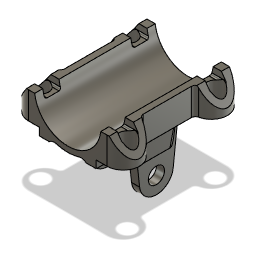
0.883.3680 - Demi-collier à chape - IGTE 21465_204886 (Autodesk Fusion 360 design; units mm, degrees)
Autodesk Fusion 360 part; units mm, degrees
sketch "Sketch1" plane through (0, 0, 0) normal (0, 0, 1) x (1, 0, 0)
  line L0 (0, 0) -> (0, -55) construction
  line L1 (-30.5, 0) -> (-30.5, -55) construction
  line L2 (30.5, 0) -> (30.5, -55) construction
  line L3 (0, 0) -> (100, 0) construction
  line L4 (0, 0) -> (-100, 0) construction
  line L5 (0, 67.5) -> (100, 67.5) construction
  line L6 (0, -67.5) -> (100, -67.5) construction
  line L7 (0, -67.5) -> (-100, -67.5) construction
  line L8 (0, -55) -> (0, -67.5) construction
  line L9 (0, -3) -> (100, -3) construction
  line L10 (0, -3) -> (-100, -3) construction
  line L11 (15, 0) -> (15, -55) construction
  line L12 (15, -55) -> (15, -67.5) construction
  line L13 (-15, 0) -> (-15, -55) construction
  line L14 (-15, -55) -> (-15, -67.5) construction
  line L15 (-15, -67.5) -> (-21, -67.5)
  arc A0 (-24.4164, -3) -> (0, -24.6) centre (0, 0) ccw
  line L16 (-30.5, -3) -> (-28.4422, -3)
  line L17 (28.4422, -3) -> (30.5, -3)
  line L18 (-30.5, -3) -> (-30.5, -23) construction
  line L19 (-30.5, -23) -> (-41, -23)
  line L20 (-41, -23) -> (-41, -18)
  line L21 (-41, -18) -> (-30.5, -3)
  line L22 (-21, -67.5) -> (-21, -22.9991)
  arc A1 (-28.4422, -3) -> (-22.9689, -17.0408) centre (0, 0) ccw
  arc A2 (-8.5119, -27.304) -> (0, -28.6) centre (0, 0) ccw
  arc A3 (-21, -22.9991) -> (-22.9689, -17.0408) centre (-31, -22.9991) ccw
  line L23 (-15, -67.5) -> (-15, -32.0774)
  arc A4 (-8.5119, -27.304) -> (-15, -32.0774) centre (-10, -32.0774) ccw
  line L24 (-24.4164, -3) -> (-28.4422, -3)
  line L25 (-30.5, -23) -> (-21, -23)
  line L26 (15, -67.5) -> (21, -67.5)
  line L27 (15, -55) -> (15, -67.5) construction
  line L28 (21, -67.5) -> (21, -22.9991)
  line L29 (15, -67.5) -> (15, -32.0774)
  arc A5 (15, -32.0774) -> (8.5119, -27.304) centre (10, -32.0774) ccw
  arc A6 (0, -28.6) -> (8.5119, -27.304) centre (0, 0) ccw
  arc A7 (0, -24.6) -> (24.4164, -3) centre (0, 0) ccw
  arc A8 (22.9689, -17.0408) -> (21, -22.9991) centre (31, -22.9991) ccw
  arc A9 (22.9689, -17.0408) -> (28.4422, -3) centre (0, 0) ccw
  line L30 (24.4164, -3) -> (28.4422, -3)
  line L31 (30.5, -3) -> (28.4422, -3)
  line L32 (41, -18) -> (30.5, -3)
  line L33 (41, -23) -> (41, -18)
  line L34 (30.5, -23) -> (41, -23)
  line L35 (30.5, -23) -> (21, -23)
  dimension "d1" = 55
  dimension "d2" = 30.5
  dimension "d3" = 30.5
  dimension "d4" = 100
  dimension "d6" = 67.5
  dimension "d7" = 3
  dimension "d8" = 15
  dimension "d9" = 15
  dimension "d11" = 6
  dimension "d14" = 24.6
  dimension "d15" = 28.6
  dimension "d19" = 20
  dimension "d20" = 10.5
  dimension "d21" = 5
  dimension "d22" = 10
  dimension "d23" = 5
  constraint coincident L0.start L3.start
  constraint symmetric L0 L3.start L4.start
  constraint symmetric L0 L3.end L4.end
  constraint parallel L3 L5
  constraint perpendicular L7 L8
  constraint coincident L9 L17.start
  constraint coincident L10 A0.start
  constraint coincident L10 L16.end
  constraint coincident L10 L16.start
  constraint coincident L1 L16.start
  constraint perpendicular L1 L16
  constraint coincident L9 L17.end
  constraint coincident L2 L17.end
  constraint perpendicular L2 L17
  constraint perpendicular L15 L22
  constraint concentric A1 A2
  constraint tangent L22 A3
  constraint tangent A1 A3
  constraint perpendicular L15 L23
  constraint tangent L23 A4
  constraint tangent A2 A4
  constraint coincident L0 A2.end
  constraint coincident L0 A0.end
  constraint perpendicular L13 L24
  constraint perpendicular L22 L25
  constraint coincident L22 L25.end
  constraint symmetric L0 L13.end L11.end
  constraint symmetric L0 L14.end L12.end
  constraint symmetric L0 L15.end L26.end
  constraint symmetric L0 A0.start A7.end
  constraint symmetric L0 A0 A7
  constraint symmetric L0 L16.end L17.start
  constraint symmetric L0 L16.start L17.end
  constraint symmetric L0 L18.end L34.start
  constraint symmetric L0 L19.end L33.start
  constraint symmetric L0 L20.end L32.start
  constraint symmetric L0 A1 A9
  constraint symmetric L0 A2 A6
  constraint symmetric L0 L22.end L28.end
  constraint symmetric L0 A1.end A8.start
  constraint symmetric L0 A3 A8
  constraint symmetric L0 L23.end L29.end
  constraint symmetric L0 A2.start A5.end
  constraint symmetric L0 A4 A5
  constraint symmetric L0 A2.end A6.start
  constraint symmetric L0 A0.end A7.start
  constraint symmetric L0 L25.end L35.end
  measures "d1" distance of L0.start L0.end
  measures "d4" distance of L0.start L3.end
  measures "d11" distance of L14.end L15.end
  measures "d14" radius of A0
  measures "d15" radius of A1
  measures "d19" distance of L16.start L18.end
  measures "d20" distance of L18.end L19.end
  measures "d21" distance of L19.end L20.end
  measures "d22" radius of A3
  measures "d23" radius of A4
extrude "Extrude1" add sketch "Sketch1" along normal mid plane 89
sketch "Sketch2" plane through (0, 0, 0) normal (1, 0, 0) x (0, 0, -1)
  line L0 (44.5, -3) -> (-44.5, -3) construction
  line L1 (0, 0) -> (0, -110) construction
  line L2 (0, 0) -> (100, 0) construction
  line L3 (0, 0) -> (-100, 0) construction
  line L4 (0, -55) -> (-100, -55) construction
  line L5 (0, -55) -> (100, -55) construction
  circle A0 centre (0, -55) radius 6
  line L6 (-44.5, -67.5) -> (-44.5, -23) construction
  line L7 (-44.5, -23) -> (-44.5, -18) construction
  line L8 (-44.5, -18) -> (-44.5, -3)
  line L9 (44.5, -3) -> (-44.5, -3) construction
  line L10 (44.5, -3) -> (44.5, -18) construction
  line L11 (44.5, -18) -> (44.5, -23) construction
  line L12 (44.5, -23) -> (44.5, -67.5) construction
  line L13 (44.5, -67.5) -> (-44.5, -67.5) construction
  arc A1 (-12.424, -56.3759) -> (12.424, -56.3759) centre (0, -55) ccw
  line L14 (44.5, -27.304) -> (-44.5, -27.304) construction
  line L15 (-44.5, -27.304) -> (-44.5, -28.6)
  line L16 (-44.5, -27.304) -> (44.5, -27.304) construction
  line L17 (44.5, -28.6) -> (44.5, -27.304)
  line L18 (-44.5, -27.304) -> (-44.5, -28.6)
  line L19 (-44.5, -28.6) -> (44.5, -28.6)
  line L20 (-15.5, 0) -> (-15.5, -110) construction
  line L21 (15.5, 0) -> (15.5, -110) construction
  line L22 (15.5, -28.6) -> (12.424, -56.3759)
  line L23 (-15.5, -28.6) -> (-12.424, -56.3759)
  line L24 (44.5, -3) -> (44.5, -28.6)
  line L25 (-44.5, -3) -> (-44.5, -28.6)
  line L26 (37, -9) -> (-31, -9) construction
  line L27 (-32.5, 0) -> (-32.5, -110) construction
  line L28 (32.5, 0) -> (32.5, -110) construction
  line L29 (21.5, -3) -> (32.5, -3)
  line L30 (32.5, -3) -> (44.5, -3) construction
  line L31 (0, -3) -> (9.5, -3)
  line L32 (0, -3) -> (-9.5, -3)
  line L33 (44.5, -28.6) -> (44.5, -67.5)
  line L34 (0, -67.5) -> (44.5, -67.5)
  line L35 (-44.5, -28.6) -> (-44.5, -67.5)
  line L36 (-44.5, -67.5) -> (0, -67.5)
  line L37 (9.5, -3) -> (21.5, -3)
  line L38 (-44.5, -3) -> (-32.5, -3)
  line L39 (-20.5, -3) -> (0, -3)
  line L40 (20.5, -3) -> (0, -3)
  line L41 (-44.5, -9) -> (31, -9) construction
  line L42 (44.5, -3) -> (32.5, -3) construction
  line L43 (32.5, -3) -> (35.5, -3) construction
  line L44 (44.5, -3) -> (-44.5, -3)
  line L45 (44.5, -3) -> (38.5, -3) construction
  line L46 (38.5, -3) -> (38.5, -7.5)
  line L47 (37, -9) -> (28, -9)
  line L48 (26.5, -7.5) -> (26.5, -3)
  arc A2 (37, -9) -> (38.5, -7.5) centre (37, -7.5) ccw
  arc A3 (26.5, -7.5) -> (28, -9) centre (28, -7.5) ccw
  line L49 (-38.5, -3) -> (-38.5, -7.5)
  arc A4 (-38.5, -7.5) -> (-37, -9) centre (-37, -7.5) ccw
  line L50 (-37, -9) -> (-28, -9)
  arc A5 (-28, -9) -> (-26.5, -7.5) centre (-28, -7.5) ccw
  line L51 (-26.5, -7.5) -> (-26.5, -3)
  point P0 (35.5, -9)
  point P1 (23.5, -9)
  point P2 (-35.5, -9)
  point P3 (-23.5, -9)
  point P4 (26.5, -9)
  dimension "d26" = 55
  dimension "d27" = 12
  dimension "d28" = 25
  dimension "d29" = 15.5
  dimension "d30" = 15.5
  dimension "d32" = 6
  dimension "d33" = 32.5
  dimension "d34" = 32.5
  dimension "d40" = 12
  dimension "d56" = 3
  dimension "d57" = 6
  dimension "d58" = 12
  dimension "d61" = 12
  dimension "d63" = 6
  dimension "d66" = 1.5
  dimension "d67" = 1.5
  constraint coincident L1.start L2.start
  constraint perpendicular L0 L1
  constraint perpendicular L1 L2
  constraint symmetric L1 L2.start L3.start
  constraint symmetric L1 L2.end L3.end
  constraint coincident L4.start L5.start
  constraint concentric A0 A1
  constraint coincident L15.end L18.end
  constraint coincident L17.start L19.end
  constraint coincident L21 L22.start
  constraint coincident L19 L22.start
  constraint tangent A1 L22
  constraint coincident L20 L23.start
  constraint coincident L19 L23.start
  constraint tangent A1 L23
  constraint coincident L0.start L9.start
  constraint coincident L0.end L8.end
  constraint coincident L9 L29.start
  constraint coincident L28 L29.end
  constraint coincident L0 L29.end
  constraint coincident L0 L31.end
  constraint midpoint L0 L31.start
  constraint symmetric L1 L31.end L32.end
  constraint symmetric L1 L31.start L32.start
  constraint coincident L12.end L13.start
  constraint midpoint L13 L34.start
  constraint coincident L6.start L13.end
  constraint tangent A1 L36
  constraint coincident L9 L39.start
  constraint symmetric L1 L0.end L0.start
  constraint coincident L41 P2
  constraint perpendicular L0 L48
  constraint coincident L0 L48.end
  constraint tangent L46 A2
  constraint tangent L26 A2
  constraint coincident P4 L47
  constraint coincident P4 L48
  constraint tangent L47 A3
  constraint tangent L48 A3
  constraint symmetric L1 L45.end L49.start
  constraint symmetric L1 L48.end L51.end
  constraint symmetric L1 L46.end L49.end
  constraint symmetric L1 L26.start A4.end
  constraint symmetric L1 A2 A4
  constraint symmetric L1 L47.end L50.end
  constraint symmetric L1 L48.start A5.end
  constraint symmetric L1 A3 A5
  measures "d27" diameter of A0
  measures "d28" diameter of A1
  measures "d32" distance of L9 L26
  measures "d40" distance of L0.end L38.end
  measures "d56" distance of L29.end L43.end
  measures "d57" distance of L43.end P0
  measures "d58" distance of P0 P1
  measures "d61" distance of P2 P3
  measures "d63" distance of L0.start L45.end
  measures "d66" radius of A2
  measures "d67" radius of A3
extrude "Extrude2" cut sketch "Sketch2" along normal through all and the other way through all contours A0 | L38 L44 L49 A4 L50 A5 L51 | A1 L19 L23 L35 L36 | A1 L19 L22 L33 L34 | L29 L44 L46 L47 L48 A2 A3
sketch "Sketch3" plane through (0, 0, 0) normal (0, 1, 0) x (1, 0, 0)
  line L0 (-41, 44.5) -> (-41, -44.5) construction
  line L1 (41, 44.5) -> (41, -44.5) construction
  line L2 (-24.4164, 44.5) -> (24.4164, 44.5) construction
  line L3 (24.4164, 44.5) -> (30.5, 44.5) construction
  line L4 (30.5, 44.5) -> (41, 44.5) construction
  line L5 (-24.4164, 44.5) -> (-30.5, 44.5) construction
  line L6 (-41, 44.5) -> (-30.5, 44.5) construction
  line L7 (-30.5, -44.5) -> (-41, -44.5) construction
  line L8 (-24.4164, -44.5) -> (-30.5, -44.5) construction
  line L9 (24.4164, -44.5) -> (-24.4164, -44.5) construction
  line L10 (30.5, -44.5) -> (24.4164, -44.5) construction
  line L11 (41, -44.5) -> (30.5, -44.5) construction
  line L12 (0, -44.5) -> (0, 44.5) construction
  line L13 (-41, 0) -> (41, 0) construction
  line L14 (29, -44.5) -> (29, -32.5) construction
  line L15 (29, -32.5) -> (41, -32.5) construction
  line L16 (41, -32.5) -> (41, -44.5) construction
  line L17 (29, 32.5) -> (41, 32.5) construction
  line L18 (29, 44.5) -> (29, 32.5) construction
  line L19 (-29, 32.5) -> (-41, 32.5) construction
  line L20 (-29, 44.5) -> (-29, 32.5) construction
  line L21 (-29, -32.5) -> (-41, -32.5) construction
  line L22 (-29, -44.5) -> (-29, -32.5) construction
  line L23 (29, -32.5) -> (29, -20.5) construction
  arc A0 (29, -44.5) -> (31.4, -20.7424) centre (29, -32.5) ccw
  arc A1 (31.4, 20.7424) -> (29, 44.5) centre (29, 32.5) ccw
  line L24 (29, 32.5) -> (29, 20.5) construction
  line L25 (-29, -32.5) -> (-29, -20.5) construction
  arc A2 (-31.4, -20.7424) -> (-29, -44.5) centre (-29, -32.5) ccw
  line L26 (-29, 32.5) -> (-29, 20.5) construction
  arc A3 (-29, 44.5) -> (-31.4, 20.7424) centre (-29, 32.5) ccw
  line L27 (-29, -17.8031) -> (-29, 17.8031)
  line L28 (29, -17.8031) -> (29, 17.8031)
  line L29 (-29, -44.5) -> (29, -44.5)
  line L30 (-29, 44.5) -> (29, 44.5)
  arc A4 (29, -17.8031) -> (31.4, -20.7424) centre (32, -17.8031) ccw
  arc A5 (31.4, 20.7424) -> (29, 17.8031) centre (32, 17.8031) ccw
  arc A6 (-31.4, -20.7424) -> (-29, -17.8031) centre (-32, -17.8031) ccw
  arc A7 (-29, 17.8031) -> (-31.4, 20.7424) centre (-32, 17.8031) ccw
  line L31 (-41, -32.5) -> (-41, 32.5)
  line L32 (41, -32.5) -> (41, 32.5)
  line L33 (41, 32.5) -> (41, 44.5)
  line L34 (29, 44.5) -> (41, 44.5)
  line L35 (-41, 32.5) -> (-41, 44.5)
  line L36 (-29, 44.5) -> (-41, 44.5)
  line L37 (-29, -44.5) -> (-41, -44.5)
  line L38 (-41, -44.5) -> (-41, -32.5)
  line L39 (41, -44.5) -> (41, -32.5)
  line L40 (29, -44.5) -> (41, -44.5)
  line L41 (29, -32.5) -> (32, -32.5)
  circle A8 centre (32, -32.5) radius 6
  circle A9 centre (32, 32.5) radius 6
  circle A10 centre (-32, 32.5) radius 6
  circle A11 centre (-32, -32.5) radius 6
  line L42 (-30.5, 38.5) -> (-24.4164, 38.5)
  dimension "d44" = 12
  dimension "d45" = 12
  dimension "d47" = 3
  dimension "d55" = 12
  constraint midpoint L9 L12.start
  constraint midpoint L2 L12.end
  constraint midpoint L0 L13.start
  constraint midpoint L1 L13.end
  constraint vertical L14
  constraint horizontal L15
  constraint vertical L16
  constraint coincident L1.end L11.start
  constraint symmetric L13 L14.start L18.start
  constraint symmetric L13 L14.end L17.start
  constraint symmetric L13 L15.end L17.end
  constraint symmetric L12 L14.start L22.start
  constraint symmetric L12 L14.end L21.start
  constraint symmetric L12 L15.end L21.end
  constraint symmetric L12 L17.start L19.start
  constraint symmetric L12 L17.end L19.end
  constraint symmetric L12 L18.start L20.start
  constraint coincident L14.end L15.start
  constraint coincident L15.end A0
  constraint perpendicular L15 L23
  constraint symmetric L13 L23.end L24.end
  constraint symmetric L13 A0 A1
  constraint symmetric L12 L23.end L25.end
  constraint symmetric L12 A0 A2
  constraint symmetric L12 L24.end L26.end
  constraint symmetric L12 A1 A3
  constraint tangent L27 A7
  constraint tangent A3 A7
  constraint equal A4 A7
  constraint coincident L1.start L4.end
  constraint coincident L0.start L6.start
  constraint coincident L0.end L7.end
  constraint coincident L41.end A8.centre
  constraint symmetric L13 A8 A9
  constraint symmetric L12 A8 A11
  constraint symmetric L12 A9 A10
  measures "d44" distance of L1.end L15.end
  measures "d45" distance of L1.end L14.start
  measures "d47" radius of A4
  measures "d55" diameter of A8
extrude "Extrude3" cut sketch "Sketch3" along normal through all and the other way through all contours A0 L39 L40 | A0 A1 L28 A4 A5 L32 | A2 L37 L38 | A1 L33 L34 | A2 A3 L27 A6 A7 L31 | A3 L35 L36 | A8 | A9 | A10 | A11
sketch "Sketch4" plane through (0, 0, 0) normal (0, 0, 1) x (1, 0, 0)
  arc A0 (-24.4164, -3) -> (24.4164, -3) centre (0, 0) ccw construction
  arc A1 (-8.5119, -27.304) -> (8.5119, -27.304) centre (0, 0) ccw construction
  line L0 (21, -67.5) -> (21, -56.3759) construction
  line L1 (15, -56.3759) -> (15, -67.5) construction
  line L2 (15, -56.3759) -> (15, -32.0774) construction
  line L3 (15, -56.3759) -> (21, -56.3759) construction
  line L4 (21, -28.6) -> (21, -56.3759) construction
  line L5 (21, -23) -> (29, -23) construction
  line L6 (21, -28.6) -> (21, -23) construction
  line L7 (29, -23) -> (41, -23) construction
  line L8 (29, -3) -> (24.4164, -3) construction
  line L9 (30.5, -3) -> (29, -3) construction
  line L10 (41, -18) -> (30.5, -3) construction
  line L11 (0, 0) -> (0, -83.2034) construction
  circle A2 centre (0, 0) radius 28.6 construction
  line L12 (15, -67.5) -> (21, -67.5) construction
  line L13 (15, -42.5) -> (21, -42.5) construction
  line L14 (21, -42.5) -> (28.0922, -5.3652)
  line L15 (21, -42.5) -> (21, -19.4155)
  arc A3 (21, -19.4155) -> (28.0922, -5.3652) centre (0, 0) ccw
  line L16 (-21, -42.5) -> (-21, -19.4155)
  arc A4 (-28.0922, -5.3652) -> (-21, -19.4155) centre (0, 0) ccw
  line L17 (-21, -42.5) -> (-28.0922, -5.3652)
  dimension "d50" = 25
  constraint coincident A0.centre A1.centre
  constraint vertical L11
  constraint concentric A0 A2
  constraint coincident L1.end L12.start
  constraint coincident L0.start L12.end
  constraint coincident A2 L14.end
  constraint tangent A2 L14
  constraint perpendicular L13 L15
  constraint coincident A2 L15.end
  constraint symmetric L11 L13.end L16.start
  constraint symmetric L11 L14.end A4.start
  constraint symmetric L11 L15.end L16.end
  constraint symmetric L11 A3 A4
extrude "Extrude4" add sketch "Sketch4" along normal mid plane 20
fillet "Fillet1" radius 4 4 edges at (21, -32.75, 10) (21, -32.75, -10) (-21, -32.75, -10) (-21, -32.75, 10)
equation "d14 = 12.30 mm * 2"
equation "d15 = ( 14.30 * 2 ) * 1 mm"
